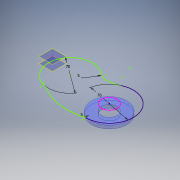
# Autodesk Inventor part: body depart
Saved by Autodesk Inventor 2018.1 (Build 221171000, 171)
## iProperties
Created: 2022-07-20
Part Number: body depart
Material: Generic
Document SubType Name: Modeling
Designer: mouta
Density: 1 g/cm^3
Appearance: Default
Author: mouta
Autodesk Inventor part; units mm, degrees
ref_plane "YZ Plane" through (0, 0, 0) normal (1, 0, 0) x (0, 1, 0)
ref_plane "XZ Plane" through (0, 0, 0) normal (0, 1, 0) x (-1, 0, 0)
ref_plane "XY Plane" through (0, 0, 0) normal (0, 0, 1) x (1, 0, 0)
ref_plane "Work Plane1" through (0, 0, 0) normal (0, 0, -1) x (-1, 0, 0)
sketch "Sketch2" plane through (0, 0, 0) normal (0, 0, -1) x (-1, 0, 0)
  circle A0 centre (-110.2989, -19.8991) radius 12.5 projected
  arc A1 (-94.6273, 14.7187) -> (-110.9661, -57.8933) centre (-110.2989, -19.8991) ccw
  arc A2 (-94.6273, 14.7187) -> (-66.2148, 12.4187) centre (-77.8689, 45.0954) ccw
  arc A3 (-33.9955, -46.3001) -> (-64.4521, 13.5018) centre (-40.3561, -11.8829) ccw
  arc A4 (-66.2148, 12.4187) -> (-64.4521, 13.5018) centre (-67.8944, 17.1282) ccw
  arc A5 (-33.9955, -46.3001) -> (-35.1369, -46.6564) centre (-33.0868, -51.2168) ccw
  arc A6 (-109.6375, -58.0974) -> (-35.1369, -46.6564) centre (-84.5507, 26.8294) ccw
  arc A7 (-109.6375, -58.0974) -> (-110.9661, -57.8933) centre (-111.0539, -62.8925) ccw
  point P0 (0, 0)
  point P1 (-110.2989, -57.8991)
  point P2 (-29.7821, -43.8025)
  dimension "d38" = 76
  dimension "d42" = 70
  dimension "d43" = 5
  dimension "d48" = 5
  constraints: 15 point on circle, 7 centre point, 5 tangent, 1 coincident, 1 equal radius
  measures "d38" diameter of A1
  measures "d42" diameter of A3
  measures "d43" radius of A4
  measures "d48" radius of A7
ref_plane "Work Plane2" through (0, 0, -10) normal (0, 0, -1) x (-1, 0, 0)
sketch "Sketch3" plane through (0, 0, -10) normal (0, 0, -1) x (-1, 0, 0)
  circle A0 centre (-110.2989, -19.8991) radius 12.5 projected
  circle A1 centre (-110.2989, -19.8991) radius 28
  circle A2 centre (-110.2989, -19.8991) radius 12.5
  point P0 (0, 0)
  dimension "d44" = 56
  dimension "d45" = 25
  constraints: 2 centre point, 2 coincident
  measures "d44" diameter of A1
  measures "d45" diameter of A2
extrude "Extrusion5" add sketch "Sketch3" along normal blind 5
body "Solid3"
